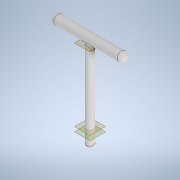
# Autodesk Inventor part: drain cover handle
Saved by Autodesk Inventor 2020.4 (Build 244396000, 396)
## iProperties
Created: 2023-07-18
Part Number: drain cover handle
Material: Generic
Document SubType Name: Modeling
Designer: Paul
Density: 1 g/cm^3
Appearance: Default
Author: Paul
Autodesk Inventor part; units mm, degrees
ref_plane "YZ Plane" through (0, 0, 0) normal (1, 0, 0) x (0, 1, 0)
ref_plane "XZ Plane" through (0, 0, 0) normal (0, 1, 0) x (-1, 0, 0)
ref_plane "XY Plane" through (0, 0, 0) normal (0, 0, 1) x (1, 0, 0)
ref_plane "Work Plane1" through (-6.35, 0, 0) normal (-1, 0, 0) x (0, 0, 1)
ref_plane "Work Plane2" through (0, 0, 0) normal (1, 0, 0) x (0, 0, -1)
sketch "Sketch3" plane through (0, 0, 0) normal (1, 0, 0) x (0, 0, -1)
  circle A0 centre (0, 0) radius 5.08
  dimension "d35" = 10.16
  constraints: 1 centre point, 1 coincident
  measures "d35" diameter of A0
extrude "Extrusion2" add sketch "Sketch3" along normal blind 101.6 and the other way blind 25.4
ref_plane "Work Plane3" through (101.6, 0, 0) normal (1, 0, 0) x (0, 0, -1)
sketch "Sketch4" plane through (101.6, 0, 0) normal (1, 0, 0) x (0, 0, -1)
  line L0 (6.35, -50.8) -> (6.35, 50.8)
  line L1 (6.35, 50.8) -> (-6.35, 50.8)
  line L2 (-6.35, 50.8) -> (-6.35, -50.8)
  line L3 (-6.35, -50.8) -> (6.35, -50.8)
  line L4 (6.35, -50.8) -> (-6.35, 50.8) construction
  line L5 (6.35, 50.8) -> (-6.35, -50.8) construction
  circle A0 centre (0, 0) radius 5.08 projected
  line L6 (0, 0) -> (0, 147.0136)
  dimension "d40" = 101.6
  dimension "d41" = 12.7
  constraints: 14 end point, 2 midpoint, 2 parallel, 2 vertical, 1 perpendicular
  measures "d40" distance of L0.start L0.end
  measures "d41" distance of L1.end L0.end
extrude "Extrusion3" add sketch "Sketch4" along normal blind 12.7 contours L3 L2 L1 L0 | A0
fillet "Fillet6" radius 6.35 4 edges at (114.3, 0, -6.35) (114.3, 0, 6.35) (101.6, 0, 6.35) (101.6, 0, -6.35)
fillet "Fillet7" radius 6.35 11 edges at (103.4599, 50.8, -4.4901) (103.4599, 50.8, 4.4901) (112.4401, 50.8, 4.4901) (112.4401, 50.8, -4.4901) (103.4599, -50.8, -4.4901) (112.4401, -50.8, -4.4901) (112.4401, -50.8, 4.4901) (103.4599, -50.8, 4.4901) (104.14, 0.0007, 5.08) (102.9018, -3.3119, -3.852) (102.9018, 3.3118, -3.8521)
fillet "Fillet8" radius 5.08 1 edges at (-25.4, 0, 5.08)
equation "\"HR\" = 7.874"
equation "\"PR\" = 5.588"
equation "\"HA\" = 55deg"
body "Solid1"
